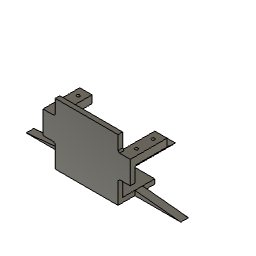
Base_Servo_Mount (Autodesk Fusion 360 design; units mm, degrees)
Autodesk Fusion 360 part; units mm, degrees
sketch "Sketch1" plane through (0, 0, 0) normal (0, 0, 1) x (1, 0, 0)
  line L0 (24.5, 21) -> (24.5, 51)
  line L1 (24.5, 51) -> (16.5, 51)
  line L2 (16.5, 51) -> (16.5, 21)
  line L3 (0, 13) -> (-30, 13)
  line L4 (-30, 13) -> (-30, 8)
  line L5 (-30, 8) -> (0, 8)
  line L6 (20.5, 51) -> (20.5, 0)
  line L7 (-30, 10.5) -> (71, 10.5)
  line L8 (71, 8) -> (41, 8)
  line L9 (41, 13) -> (71, 13)
  line L10 (71, 13) -> (71, 8)
  line L11 (41, 21) -> (24.5, 21)
  line L12 (16.5, 21) -> (0, 21)
  line L13 (41, 0) -> (41, 8)
  line L14 (41, 13) -> (41, 21)
  line L15 (0, 21) -> (0, 13)
  line L16 (0, 8) -> (0, 0)
  line L17 (0, 0) -> (41, 0)
  dimension "d1" = 21
  dimension "d2" = 41
  dimension "d3" = 8
  dimension "d4" = 5
  dimension "d5" = 8
  dimension "d6" = 16.5
  dimension "d7" = 20.5
  dimension "d8" = 10.5
  dimension "d10" = 30
  dimension "d42" = 30
  constraint horizontal L17
  constraint vertical L13
  constraint horizontal L11
  constraint vertical L15
  constraint coincident L16.end L17.start
  constraint vertical L0
  constraint horizontal L1
  constraint vertical L2
  constraint coincident L2.end L11
  constraint horizontal L3
  constraint vertical L4
  constraint horizontal L5
  constraint perpendicular L6 L17
  constraint perpendicular L7 L13
  constraint symmetric L3.start L6 L9.start
  constraint symmetric L3.end L6 L9.end
  constraint symmetric L4.end L6 L8.start
  constraint symmetric L5.end L6 L8.end
  constraint collinear L11 L12
  constraint collinear L13 L14
  constraint collinear L15 L16
  constraint coincident L4 L7.start
  constraint coincident L10 L7.end
  constraint coincident L1 L6.start
  measures "d1" distance of L16.end L12.end
  measures "d2" distance of L16.end L13.start
  measures "d3" distance of L3 L11
  measures "d4" distance of L3.end L4.end
  measures "d5" distance of L0 L2
  measures "d6" distance of L2 L15
  measures "d7" distance of L6 L15
  measures "d8" distance of L7 L17
  measures "d10" distance of L1 L11
  measures "d42" distance of L4 L15
extrude "Extrude1" add sketch "Sketch1" along normal blind 3
sketch "Sketch2" plane through (24.5, 0, 0) normal (1, 0, 0) x (0, 1, 0)
  line L0 (-20, 0) -> (0, 0)
  line L1 (0, 0) -> (0, 3)
  line L2 (0, 3) -> (-20, 3)
  line L3 (-20, 3) -> (-20, 0)
  line L4 (-20, 0) -> (0, 3)
  line L5 (41, 0) -> (21, 5)
  constraint coincident L0.start L3.end
  constraint coincident L1.end L2.start
extrude "Extrude2" cut sketch "Sketch2" against normal blind 8 contours L2 L3 L4
sketch "Sketch3" plane through (24.5, 0, 0) normal (1, 0, 0) x (0, 1, 0)
  line L0 (21, 0) -> (51, 0)
  line L1 (51, 0) -> (51, 3)
  line L2 (51, 3) -> (21, 3)
  line L3 (21, 3) -> (21, 0)
  line L4 (21, 3) -> (51, 0)
  constraint coincident L2.end L3.start
  constraint coincident L0.end L1.start
extrude "Extrude3" cut sketch "Sketch3" against normal blind 8 contours L1 L2 L4
sketch "Sketch4" plane through (0, 13, 0) normal (0, 1, 0) x (-1, 0, 0)
  line L0 (-71, 0) -> (-41, 0)
  line L1 (-41, 0) -> (-41, 3)
  line L2 (-41, 3) -> (-71, 3)
  line L3 (-71, 3) -> (-71, 0)
  line L4 (20, 0) -> (0, 5)
  line L5 (-71, 0) -> (-41, 3)
  constraint coincident L0.start L3.end
  constraint coincident L1.end L2.start
sketch "Sketch5" plane through (0, 13, 0) normal (0, 1, 0) x (-1, 0, 0)
extrude "Extrude4" cut sketch "Sketch4" against normal blind 5 contours L2 L3 L5
sketch "Sketch6" plane through (0, 13, 0) normal (0, 1, 0) x (-1, 0, 0)
  line L0 (0, 0) -> (30, 0)
  line L1 (30, 0) -> (30, 3)
  line L2 (30, 3) -> (0, 3)
  line L3 (0, 3) -> (0, 0)
  line L4 (0, 3) -> (30, 0)
  constraint coincident L2.end L3.start
  constraint coincident L0.end L1.start
extrude "Extrude5" cut sketch "Sketch6" against normal blind 5 contours L1 L2 L4
sketch "Sketch7" plane through (0, 0, 0) normal (0, 0, -1) x (1, 0, 0)
  line L0 (0, 0) -> (0, -8)
  line L1 (0, -8) -> (-30, -8)
  line L2 (-30, -8) -> (-30, -13)
  line L3 (-30, -13) -> (0, -13)
  line L4 (0, -13) -> (0, -21)
  line L5 (0, -21) -> (16.5, -21)
  line L6 (16.5, -21) -> (16.5, -51)
  line L7 (16.5, -51) -> (24.5, -51)
  line L8 (24.5, -51) -> (24.5, -21)
  line L9 (24.5, -21) -> (41, -21)
  line L10 (41, -21) -> (41, -13)
  line L11 (41, -13) -> (71, -13)
  line L12 (71, -13) -> (71, -8)
  line L13 (71, -8) -> (41, -8)
  line L14 (41, -8) -> (41, 0)
  line L15 (41, 0) -> (0, 0)
  line L16 (0, 0) -> (41, 0)
  line L17 (41, 0) -> (41, 3)
  line L18 (41, 3) -> (0, 3)
  line L19 (0, 3) -> (0, 0)
  dimension "d23" = 3
  constraint horizontal L16
  constraint vertical L17
  constraint horizontal L18
  constraint vertical L19
  constraint coincident L0.start L15.end
  measures "d23" distance of L14.end L17.end
extrude "Extrude6" add sketch "Sketch7" against normal blind 40 contours L15 L16 L17 L18 L19
sketch "Sketch8" plane through (0, -3, 0) normal (0, -1, 0) x (1, 0, 0)
  line L0 (0, 0) -> (41, 0)
  line L1 (41, 0) -> (41, 40)
  line L2 (41, 40) -> (0, 40)
  line L3 (0, 40) -> (0, 0)
  line L4 (41, 15) -> (49, 15)
  line L5 (49, 15) -> (49, 30)
  line L6 (49, 30) -> (41, 30)
  line L7 (41, 30) -> (41, 15)
  line L8 (20.5, 40) -> (20.5, 3)
  line L9 (0, 15) -> (-8, 15)
  line L10 (-8, 15) -> (-8, 30)
  line L11 (-8, 30) -> (0, 30)
  line L12 (0, 3) -> (41, 3)
  line L13 (0, 3) -> (41, 3)
  line L14 (0, 3) -> (41, 3)
  line L15 (0, 3) -> (41, 3)
  dimension "d24" = 15
  dimension "d25" = 27
  dimension "d28" = 8
  constraint horizontal L4
  constraint vertical L5
  constraint horizontal L6
  constraint vertical L7
  constraint coincident L1 L4.start
  constraint midpoint L2 L8.start
  constraint symmetric L4.start L8 L9.start
  constraint symmetric L4.end L8 L9.end
  constraint symmetric L5.end L8 L10.end
  constraint symmetric L6.end L8 L11.end
  measures "d24" distance of L4.end L5.end
  measures "d25" distance of L6 L12.end
  measures "d28" distance of L4.start L4.end
extrude "Extrude7" add sketch "Sketch8" against normal up to surface (3 mm away) contours L3 L9 L10 L11 | L1 L4 L5 L6 L7
sketch "Sketch9" plane through (0, 0, 0) normal (0, 1, 0) x (-1, 0, 0)
  line L0 (-41, 3) -> (0, 3)
  line L1 (0, 3) -> (0, 15)
  line L2 (0, 15) -> (8, 15)
  line L3 (8, 15) -> (8, 30)
  line L4 (8, 30) -> (0, 30)
  line L5 (0, 30) -> (0, 40)
  line L6 (0, 40) -> (-41, 40)
  line L7 (-41, 40) -> (-41, 30)
  line L8 (-41, 30) -> (-49, 30)
  line L9 (-49, 30) -> (-49, 15)
  line L10 (-49, 15) -> (-41, 15)
  line L11 (-41, 15) -> (-41, 3)
  line L12 (-49, 30) -> (-41, 30)
  line L13 (-41, 30) -> (-41, 25)
  line L14 (-41, 25) -> (-49, 25)
  line L15 (-49, 25) -> (-49, 30)
  line L16 (8, 30) -> (0, 30)
  line L17 (0, 30) -> (0, 25)
  line L18 (0, 25) -> (8, 25)
  line L19 (8, 25) -> (8, 30)
  dimension "d29" = 5
  dimension "d43" = 5
  constraint horizontal L12
  constraint vertical L13
  constraint horizontal L14
  constraint vertical L15
  constraint coincident L8.end L9.start
  constraint horizontal L16
  constraint vertical L17
  constraint horizontal L18
  constraint vertical L19
  constraint coincident L3.end L4.start
  measures "d29" distance of L7.end L13.end
  measures "d43" distance of L4.end L17.end
extrude "Extrude8" add sketch "Sketch9" along normal up to surface (21 mm away) contours L8 L9 L12 L13 L14 L15 | L3 L4 L16 L17 L18 L19
sketch "Sketch10" plane through (0, 0, 30) normal (0, 0, 1) x (-1, 0, 0)
  line L0 (8, -21) -> (8, 3)
  line L1 (8, 3) -> (0, 3)
  line L2 (0, 3) -> (0, 0)
  line L3 (0, 0) -> (0, -21)
  line L4 (0, -21) -> (8, -21)
  circle A0 centre (4, -16) radius 1
  circle A1 centre (4, -5) radius 1
  circle A2 centre (-45, -16) radius 1
  circle A3 centre (-45, -5) radius 1
  line L5 (-41, 0) -> (-41, -21)
  line L6 (0, 0) -> (-41, 0)
  dimension "d32" = 2
  dimension "d33" = 5
  dimension "d34" = 4
  dimension "d36" = 4
  dimension "d39" = 5
  constraint equal A0 A1
  constraint equal A0 A2
  constraint equal A0 A3
  constraint vertical A0.centre A1.centre
  constraint horizontal A0.centre A2.centre
  constraint horizontal A1.centre A3.centre
  constraint vertical A2.centre A3.centre
  measures "d32" diameter of A0
  measures "d33" distance of L4 A0.centre
  measures "d34" distance of L3 A0.centre
  measures "d36" distance of A2.centre L5
  measures "d39" distance of A1.centre L6
extrude "Extrude9" cut sketch "Sketch10" against normal blind 5 contours A0 | A1 | A2 | A3
chamfer "Chamfer1" distance 1 angle 45 2 edges at (-4, 0, 25) (45, 0, 25)
chamfer "Chamfer2" distance 1 angle 45 4 edges at (0, -1.5, 15) (41, -1.5, 15) (41, -1.5, 30) (0, -1.5, 30)
equation "d6 = ( ( 41 - 8 ) / 2 ) * 1 mm"
equation "d7 = ( 41 / 2 ) * 1 mm"
equation "d8 = ( 21 / 2 ) * 1 mm"
